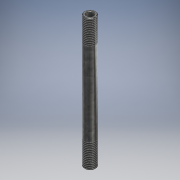
# Autodesk Inventor part: EjeManzanaD
Saved by Autodesk Inventor 2017 (Build 210142000, 142)
## iProperties
Created: 2016-06-28
Part Number: EjeManzanaD
Material: Steel
Document SubType Name: Modeling
Designer: YeseF
Density: 7.85 g/cm^3
Appearance: Steel Galvanized
Author: YeseF
Autodesk Inventor part; units mm, degrees
ref_plane "YZ Plane" through (0, 0, 0) normal (1, 0, 0) x (0, 1, 0)
ref_plane "XZ Plane" through (0, 0, 0) normal (0, 1, 0) x (-1, 0, 0)
ref_plane "XY Plane" through (0, 0, 0) normal (0, 0, 1) x (1, 0, 0)
sketch "Sketch1" plane through (0, 0, 0) normal (0, 0, 1) x (1, 0, 0)
  circle A0 centre (0, 0) radius 4.5
  circle A1 centre (0, 0) radius 2.56
  dimension "d0" = 9
  dimension "d1" = 5.12
  constraints: 2 centre point, 2 coincident
  measures "d0" diameter of A0
  measures "d1" diameter of A1
extrude "Extrusion1" add sketch "Sketch1" along normal blind 108.2
thread "Thread1" size "M9x1.25" class "6g" standard "ANSI Metric M Profile" length 20
ref_plane "Work Plane1" through (0, 0, 54.1) normal (0, 0, 1) x (1, 0, 0)
thread "Thread2" size "M9x1.25" class "6g" standard "ANSI Metric M Profile" length 20
chamfer "Chamfer2" distance 0.5 angle 45 4 edges at (-2.56, 0, 108.2) (-4.5, 0, 108.2) (-4.5, 0, 0) (-2.56, 0, 0)
body "Solid1"
